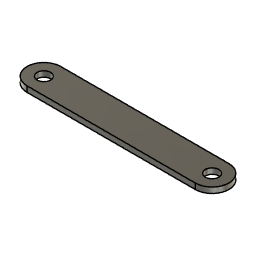
upper leg v0 (Autodesk Fusion 360 design; units mm, degrees)
Autodesk Fusion 360 part; units mm, degrees
sketch "Sketch1" plane through (0, 0, 0) normal (0, 0, 1) x (1, 0, 0)
  line L0 (0, -15) -> (150, -15)
  arc A0 (150, -15) -> (150, 15) centre (150, 0) ccw
  line L1 (150, 15) -> (0, 15)
  arc A1 (0, 15) -> (0, -15) centre (0, 0) ccw
  line L2 (0, 0) -> (150, 0) construction
  circle A2 centre (0, 0) radius 6
  circle A3 centre (150, 0) radius 6
  dimension "d1" = 150
  dimension "d2" = 30
  dimension "d3" = 12
  dimension "d4" = 12
  constraint tangent L0 A0
  constraint tangent A0 L1
  constraint parallel L0 L1
  constraint tangent L1 A1
  constraint tangent L0 A1
  constraint horizontal L2
  constraint coincident A1.centre L2.start
  constraint concentric A1 A2
  constraint concentric A0 A3
  measures "d1" distance of A0.end L1.end
  measures "d2" distance of L0 L1
  measures "d3" diameter of A2
  measures "d4" diameter of A3
extrude "Extrude1" add sketch "Sketch1" along normal blind 5
